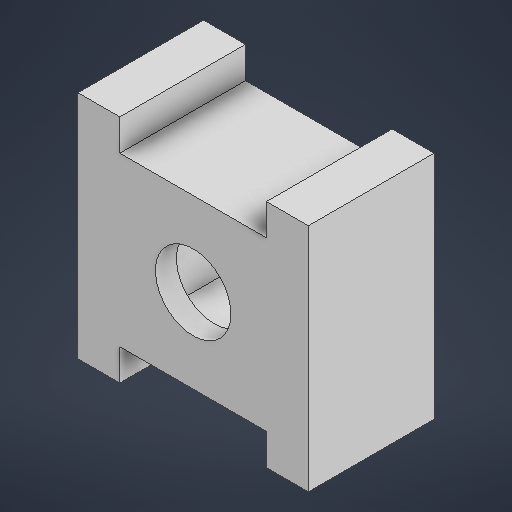
# Autodesk Inventor part: Part14
Saved by Autodesk Inventor 2027.1 (Build 311270010, 270A)
## iProperties
Created: 2026-10-10
Part Number: Part14
Material: Generic
Document SubType Name: Modeling
Designer: daniel
Density: 1 g/cm^3
Appearance: Default
Author: daniel
Autodesk Inventor part; units mm, degrees
ref_plane "YZ Plane" through (0, 0, 0) normal (1, 0, 0) x (0, 1, 0)
ref_plane "XZ Plane" through (0, 0, 0) normal (0, 1, 0) x (-1, 0, 0)
ref_plane "XY Plane" through (0, 0, 0) normal (0, 0, 1) x (1, 0, 0)
sketch "Sketch1" plane through (0, 0, 0) normal (0, 0, 1) x (1, 0, 0)
  line L0 (0, 0) -> (55, 0)
  line L1 (55, 0) -> (55, 55)
  line L2 (55, 55) -> (0, 55)
  line L3 (0, 55) -> (0, 0)
  line L4 (55, 0) -> (0, 0)
  line L5 (0, 0) -> (0, 10)
  line L6 (0, 10) -> (55, 10)
  line L7 (55, 10) -> (55, 0)
  line L8 (55, 55) -> (0, 55)
  line L9 (0, 55) -> (0, 45)
  line L10 (0, 45) -> (55, 45)
  line L11 (55, 45) -> (55, 55)
  circle A0 centre (27.5, 27.5) radius 15
  line L12 (0, 55) -> (10, 55)
  line L13 (10, 55) -> (10, 0)
  line L14 (10, 0) -> (0, 0)
  line L15 (0, 0) -> (0, 55)
  line L16 (55, 55) -> (45, 55)
  line L17 (45, 55) -> (45, 0)
  line L18 (45, 0) -> (55, 0)
  line L19 (55, 0) -> (55, 55)
  line L20 (7.5, 47.5) -> (47.5, 47.5)
  line L21 (47.5, 47.5) -> (47.5, 7.5)
  line L22 (47.5, 7.5) -> (7.5, 7.5)
  line L23 (7.5, 7.5) -> (7.5, 47.5)
  line L24 (7.5, 47.5) -> (47.5, 7.5) construction
  line L25 (47.5, 47.5) -> (7.5, 7.5) construction
  circle A1 centre (27.5, 27.5) radius 9
  point P0 (10, 0)
  point P1 (10, 10)
  point P2 (45, 10)
  point P3 (45, 45)
  point P4 (10, 45)
  point P5 (45, 47.5)
  point P6 (10, 47.5)
  point P7 (10, 7.5)
  point P8 (45, 7.5)
  dimension "d0" = 55
  dimension "d1" = 55
  dimension "d2" = 10
  dimension "d3" = 10
  dimension "d4" = 30
  dimension "d5" = 10
  dimension "d6" = 10
  dimension "d11" = 40
  dimension "d12" = 40
  dimension "d13" = 18
  constraints: 52 end point, 12 parallel, 6 horizontal, 6 perpendicular, 4 point on line, 2 centre point, 2 midpoint, 1 coincident
  measures "d0" distance of L2.end L1.end
  measures "d1" distance of L1.end L0.end
  measures "d2" distance of L4.end L5.end
  measures "d3" distance of L9.end L8.end
  measures "d4" diameter of A0
  measures "d5" distance of L18.end L17.end
  measures "d6" distance between parallel lines of L3 L13
  measures "d11" distance of L21.end L22.end
  measures "d12" distance of L20.end L21.end
  measures "d13" diameter of A1
extrude "Extrusion3" add sketch "Sketch1" against normal blind 5 contours L13 L10 L17 L6 | A0
extrude "Extrusion4" add sketch "Sketch1" against normal blind 30 contours L3 L6 L23 L22 L13 L0 | L3 L10 L23 L6 | L17 L22 L21 L6 L1 L0 | L22 L23 L6 L13 | L13 L6 L17 L22 | L3 L2 L13 L20 L23 L10 | L23 L10 L13 L6 | L17 L6 L21 L22 | L23 L20 L13 L10 | L6 L21 L10 L1 | L17 L10 L21 L6 | L13 L20 L17 L10 | L10 L21 L20 L17 L2 L1 | L17 L20 L21 L10
body "Solid2"
